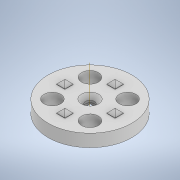
# Autodesk Inventor part: dent
Saved by Autodesk Inventor 2020 (Build 240168000, 168)
## iProperties
Created: 2020-06-16
Part Number: dent
Material: Generic
Document SubType Name: Modeling
Designer: Admin
Density: 1 g/cm^3
Appearance: Default
Author: Admin
Autodesk Inventor part; units mm, degrees
ref_plane "YZ Plane" through (0, 0, 0) normal (1, 0, 0) x (0, 1, 0)
ref_plane "XZ Plane" through (0, 0, 0) normal (0, 1, 0) x (-1, 0, 0)
ref_plane "XY Plane" through (0, 0, 0) normal (0, 0, 1) x (1, 0, 0)
sketch "Sketch1" plane through (0, 0, 0) normal (0, 1, 0) x (-1, 0, 0)
  circle A0 centre (0, 0) radius 10
  dimension "d0" = 20
  constraints: 1 centre point, 1 coincident
  measures "d0" diameter of A0
extrude "Extrusion1" add sketch "Sketch1" along normal blind 3
sketch "Sketch2" plane through (0, 3, 0) normal (0, 1, 0) x (1, 0, 0)
  line L0 (-7, -1) -> (-5, -1)
  line L1 (-5, -1) -> (-5, 1)
  line L2 (-5, 1) -> (-7, 1)
  line L3 (-7, 1) -> (-7, -1)
  point P0 (0, 0)
  dimension "d3" = 2
  dimension "d4" = 2
  dimension "d5" = 5
  dimension "d6" = 1
  constraints: 8 end point, 2 parallel, 1 horizontal, 1 perpendicular
  measures "d3" distance of L2.end L0.start
  measures "d4" distance of L1.end L2.end
  measures "d5" distance from line of L1 point (0, 0)
  measures "d6" distance from line of point (0, 0) L0
extrude "Extrusion2" add sketch "Sketch2" along normal blind 1
pattern_circular "Circular Pattern2" count 4 over 360 about axis through (0, 0, 0) along (0, 1, 0) of "Extrusion2"
chamfer "Chamfer3" distance 0.9 angle 45 16 edges at (-6, 4, 1) (-5, 4, 0) (-6, 4, -1) (-7, 4, 0) (0, 4, -5) (-1, 4, -6) (0, 4, -7) (1, 4, -6) (6, 4, -1) (7, 4, 0) (5, 4, 0) (6, 4, 1) (1, 4, 6) (-1, 4, 6) (0, 4, 5) (0, 4, 7)
sketch "Sketch3" plane through (0, 3, 0) normal (0, 1, 0) x (1, 0, 0)
  circle A0 centre (-4.5, -4.5) radius 2
  point P0 (0, 0)
  dimension "d24" = 4
  dimension "d25" = 4.5
  dimension "d26" = 4.5
  constraints: 1 centre point
  measures "d24" diameter of A0
  measures "d25" horizontal distance of point (0, 0) A0.centre
  measures "d26" horizontal distance of point (0, 0) A0.centre
extrude "Extrusion3" cut sketch "Sketch3" against normal through all
pattern_circular "Circular Pattern3" count 4 over 360 about axis through (0, 0, 0) along (0, 1, 0) of "Extrusion3"
sketch "Sketch5" plane through (0, 0, 0) normal (0, -1, 0) x (1, 0, 0)
  line L0 (-2, -2) -> (2, -2)
  line L1 (2, -2) -> (2, 2)
  line L2 (2, 2) -> (-2, 2)
  line L3 (-2, 2) -> (-2, -2)
  point P0 (0, 0)
  dimension "d39" = 4
  dimension "d40" = 4
  dimension "d41" = 2
  dimension "d42" = 2
  constraints: 8 end point, 2 parallel, 1 horizontal, 1 perpendicular
  measures "d39" distance of L2.end L0.start
  measures "d40" distance of L0.start L0.end
  measures "d41" distance from line of point (0, 0) L3
  measures "d42" distance from line of point (0, 0) L0
extrude "Extrusion5" cut sketch "Sketch5" against normal blind 1.5
sketch "Sketch6" plane through (0, 3, 0) normal (0, 1, 0) x (1, 0, 0)
  circle A0 centre (0, 0) radius 1.05
  dimension "d45" = 2.1
  constraints: 1 centre point, 1 coincident
  measures "d45" diameter of A0
extrude "Extrusion6" cut sketch "Sketch6" against normal through all
chamfer "Chamfer4" distance 1 angle 45 1 edges at (-1.05, 3, 0)
body "Solid1"
